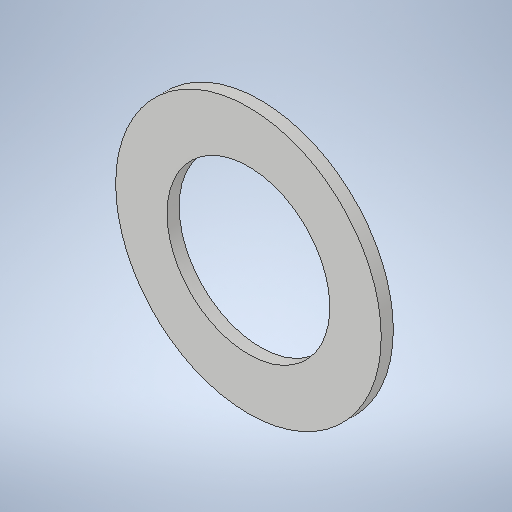
# Autodesk Inventor part: Fixierplatte_Innenring58,2mm
Saved by Autodesk Inventor 2025 (Build 290162000, 162)
## iProperties
Created: 2020-01-21
Part Number: Fixierplatte_Innenring58,2mm
Material: Generisch
Document SubType Name: Modeling
Designer: maxse
Density: 1 g/cm^3
Appearance: Vorgabe
Author: maxse
Autodesk Inventor part; units mm, degrees
(part 1 of 2)
ref_plane "YZ Plane" through (0, 0, 0) normal (1, 0, 0) x (0, 1, 0)
ref_plane "XZ Plane" through (0, 0, 0) normal (0, 1, 0) x (-1, 0, 0)
ref_plane "XY Plane" through (0, 0, 0) normal (0, 0, 1) x (1, 0, 0)
sketch "Skizze1" plane through (0, 0, 0) normal (0, 1, 0) x (-1, 0, 0)
  circle A0 centre (0, 0) radius 26.94
  circle A1 centre (0, 0) radius 43.95
  dimension "d0" = 53.88
  dimension "d1" = 87.9
  constraints: 2 centre point, 2 coincident
  measures "d0" diameter of A0
  measures "d1" diameter of A1
extrude "Extrusion1" add sketch "Skizze1" along normal blind 4
sketch "Skizze2" plane through (0, 4, 0) normal (0, 1, 0) x (1, 0, 0)
  circle A0 centre (0, 0) radius 26.94 projected
  spline S0 degree 2 poles (24.5434, -20.262) (24.7807, -19.9746) (25.3421, -19.6446) (25.6382, -19.6106) knots 0 0 0 1 2 2 2
  spline S1 degree 2 poles (25.6382, -19.6106) (25.9286, -19.5771) (26.4928, -19.7592) (26.7334, -19.9578) knots 0 0 0 1 2 2 2
  spline S2 degree 2 poles (26.7334, -19.9578) (27.0459, -20.2157) (27.2948, -20.9834) (27.1879, -21.4311) knots 0 0 0 1 2 2 2
  line L0 (27.1879, -21.4311) -> (27.2035, -21.444)
  spline S3 degree 2 poles (27.2035, -21.444) (27.6039, -21.2964) (28.2246, -21.3465) (28.5183, -21.5889) knots 0 0 0 1 2 2 2
  spline S4 degree 2 poles (28.5183, -21.5889) (28.9526, -21.9475) (28.9921, -23.0835) (28.5742, -23.5897) knots 0 0 0 1 2 2 2
  spline S5 degree 2 poles (28.5742, -23.5897) (28.1408, -24.1146) (27.0673, -24.2949) (26.6361, -23.9389) knots 0 0 0 1 2 2 2
  spline S6 degree 2 poles (26.6361, -23.9389) (26.3767, -23.7248) (26.1207, -23.0038) (26.2117, -22.6008) knots 0 0 0 1 2 2 2
  line L1 (26.2117, -22.6008) -> (26.1961, -22.5879)
  spline S7 degree 2 poles (26.1961, -22.5879) (25.7613, -22.7964) (25.025, -22.7718) (24.6688, -22.4777) knots 0 0 0 1 2 2 2
  spline S8 degree 2 poles (24.6688, -22.4777) (24.1751, -22.0702) (24.0997, -20.7995) (24.5434, -20.262) knots 0 0 0 1 2 2 2
  spline S9 degree 2 poles (25.0573, -21.9053) (25.2948, -22.1013) (25.7308, -22.146) (26.0938, -21.9991) knots 0 0 0 1 2 2 2
  spline S10 degree 2 poles (26.0938, -21.9991) (26.216, -21.9528) (26.5741, -21.7546) (26.8013, -21.6321) knots 0 0 0 1 2 2 2
  spline S11 degree 2 poles (26.8013, -21.6321) (26.8361, -21.3036) (26.6057, -20.7298) (26.3401, -20.5106) knots 0 0 0 1 2 2 2
  spline S12 degree 2 poles (26.3401, -20.5106) (25.9902, -20.2216) (25.1857, -20.2668) (24.9226, -20.5856) knots 0 0 0 1 2 2 2
  spline S13 degree 2 poles (24.9226, -20.5856) (24.6543, -20.9105) (24.7199, -21.6267) (25.0573, -21.9053) knots 0 0 0 1 2 2 2
  spline S14 degree 2 poles (27.0477, -23.4276) (27.307, -23.6417) (27.9402, -23.5812) (28.1956, -23.2718) knots 0 0 0 1 2 2 2
  spline S15 degree 2 poles (28.1956, -23.2718) (28.4277, -22.9906) (28.4151, -22.3759) (28.1495, -22.1566) knots 0 0 0 1 2 2 2
  spline S16 degree 2 poles (28.1495, -22.1566) (27.9589, -21.9993) (27.5411, -21.9644) (27.2826, -22.061) knots 0 0 0 1 2 2 2
  spline S17 degree 2 poles (27.2826, -22.061) (27.1744, -22.103) (26.7479, -22.3078) (26.5932, -22.4061) knots 0 0 0 1 2 2 2
  spline S18 degree 2 poles (26.5932, -22.4061) (26.5793, -22.7729) (26.8133, -23.2341) (27.0477, -23.4276) knots 0 0 0 1 2 2 2
  line L2 (23.8426, -27.2751) -> (22.4675, -22.7082)
  line L3 (22.4675, -22.7082) -> (22.9828, -22.2151)
  line L4 (22.9828, -22.2151) -> (24.3821, -26.9832)
  line L5 (24.3821, -26.9832) -> (26.247, -25.1988)
  line L6 (26.247, -25.1988) -> (26.6532, -25.6234)
  line L7 (26.6532, -25.6234) -> (24.3608, -27.8167)
  line L8 (24.3608, -27.8167) -> (23.8426, -27.2751)
  line L9 (19.5753, -25.2414) -> (20.2031, -24.7419)
  line L10 (20.2031, -24.7419) -> (20.7985, -25.4902)
  line L11 (20.7985, -25.4902) -> (20.1707, -25.9897)
  line L12 (20.1707, -25.9897) -> (19.5753, -25.2414)
  spline S19 degree 2 poles (17.1267, -28.864) (16.9289, -28.5626) (16.784, -27.9209) (16.8357, -27.6156) knots 0 0 0 1 2 2 2
  spline S20 degree 2 poles (16.8357, -27.6156) (16.8873, -27.3103) (17.2678, -26.7455) (17.593, -26.5321) knots 0 0 0 1 2 2 2
  spline S21 degree 2 poles (17.593, -26.5321) (17.8911, -26.3365) (18.5605, -26.0862) (18.8428, -26.0511) knots 0 0 0 1 2 2 2
  line L13 (18.8428, -26.0511) -> (19.2319, -26.6439)
  line L14 (19.2319, -26.6439) -> (19.1912, -26.6706)
  spline S22 degree 2 poles (19.1912, -26.6706) (19.0957, -26.6654) (18.7752, -26.7013) (18.594, -26.7427) knots 0 0 0 1 2 2 2
  spline S23 degree 2 poles (18.594, -26.7427) (18.3902, -26.7941) (18.0736, -26.9098) (17.9008, -27.0232) knots 0 0 0 1 2 2 2
  spline S24 degree 2 poles (17.9008, -27.0232) (17.7314, -27.1343) (17.493, -27.4653) (17.4646, -27.673) knots 0 0 0 1 2 2 2
  spline S25 degree 2 poles (17.4646, -27.673) (17.4418, -27.8672) (17.5513, -28.2703) (17.698, -28.4939) knots 0 0 0 1 2 2 2
  spline S26 degree 2 poles (17.698, -28.4939) (17.8448, -28.7175) (18.1535, -28.922) (18.3309, -28.9413) knots 0 0 0 1 2 2 2
  spline S27 degree 2 poles (18.3309, -28.9413) (18.5184, -28.9684) (18.9285, -28.8253) (19.1419, -28.6852) knots 0 0 0 1 2 2 2
  spline S28 degree 2 poles (19.1419, -28.6852) (19.3722, -28.5341) (19.7829, -28.1628) (19.9017, -28.0411) knots 0 0 0 1 2 2 2
  line L15 (19.9017, -28.0411) -> (21.3157, -30.1955)
  line L16 (21.3157, -30.1955) -> (19.0224, -31.7007)
  line L17 (19.0224, -31.7007) -> (18.7001, -31.2095)
  line L18 (18.7001, -31.2095) -> (20.4548, -30.0579)
  line L19 (20.4548, -30.0579) -> (19.7233, -28.9434)
  spline S29 degree 2 poles (19.7233, -28.9434) (19.6306, -29.0236) (19.4408, -29.1628) (19.3595, -29.2161) knots 0 0 0 1 2 2 2
  spline S30 degree 2 poles (19.3595, -29.2161) (19.0377, -29.4273) (18.525, -29.6136) (18.2195, -29.5911) knots 0 0 0 1 2 2 2
  spline S31 degree 2 poles (18.2195, -29.5911) (17.9106, -29.5709) (17.3757, -29.2434) (17.1267, -28.864) knots 0 0 0 1 2 2 2
  line L20 (11.7152, -29.7699) -> (12.6245, -31.7422)
  spline S32 degree 2 poles (12.6245, -31.7422) (12.7331, -31.9777) (12.9548, -32.3618) (13.0646, -32.4451) knots 0 0 0 1 2 2 2
  spline S33 degree 2 poles (13.0646, -32.4451) (13.1794, -32.5394) (13.4582, -32.5536) (13.6532, -32.4637) knots 0 0 0 1 2 2 2
  spline S34 degree 2 poles (13.6532, -32.4637) (13.8298, -32.3823) (14.1345, -31.9786) (14.2529, -31.6741) knots 0 0 0 1 2 2 2
  spline S35 degree 2 poles (14.2529, -31.6741) (14.2255, -31.6243) (14.1519, -31.4842) (14.1078, -31.3885) knots 0 0 0 1 2 2 2
  line L21 (14.1078, -31.3885) -> (13.073, -29.1439)
  line L22 (13.073, -29.1439) -> (13.647, -28.8793)
  line L23 (13.647, -28.8793) -> (14.5563, -30.8516)
  spline S36 degree 2 poles (14.5563, -30.8516) (14.6649, -31.0871) (14.8866, -31.4712) (14.9964, -31.5544) knots 0 0 0 1 2 2 2
  spline S37 degree 2 poles (14.9964, -31.5544) (15.1112, -31.6487) (15.39, -31.663) (15.585, -31.5731) knots 0 0 0 1 2 2 2
  spline S38 degree 2 poles (15.585, -31.5731) (15.769, -31.4882) (16.0705, -31.0681) (16.1787, -30.7996) knots 0 0 0 1 2 2 2
  line L24 (16.1787, -30.7996) -> (15.0048, -28.2533)
  line L25 (15.0048, -28.2533) -> (15.5788, -27.9887)
  line L26 (15.5788, -27.9887) -> (17.1497, -31.396)
  line L27 (17.1497, -31.396) -> (16.5757, -31.6606)
  line L28 (16.5757, -31.6606) -> (16.4027, -31.2853)
  spline S39 degree 2 poles (16.4027, -31.2853) (16.2817, -31.6133) (15.9538, -32.0634) (15.6889, -32.1855) knots 0 0 0 1 2 2 2
  spline S40 degree 2 poles (15.6889, -32.1855) (15.3872, -32.3246) (14.7926, -32.2641) (14.527, -32.0073) knots 0 0 0 1 2 2 2
  spline S41 degree 2 poles (14.527, -32.0073) (14.3997, -32.4185) (14.0441, -32.9438) (13.7571, -33.0762) knots 0 0 0 1 2 2 2
  spline S42 degree 2 poles (13.7571, -33.0762) (13.5363, -33.1779) (13.1129, -33.208) (12.9092, -33.1146) knots 0 0 0 1 2 2 2
  spline S43 degree 2 poles (12.9092, -33.1146) (12.7018, -33.0228) (12.3372, -32.6287) (12.176, -32.2792) knots 0 0 0 1 2 2 2
  line L29 (12.176, -32.2792) -> (11.1412, -30.0346)
  line L30 (11.1412, -30.0346) -> (11.7152, -29.7699)
  line L31 (6.1873, -31.3881) -> (6.7283, -33.4915)
  spline S44 degree 2 poles (6.7283, -33.4915) (6.7928, -33.7426) (6.9421, -34.1602) (7.0351, -34.2618) knots 0 0 0 1 2 2 2
  spline S45 degree 2 poles (7.0351, -34.2618) (7.1312, -34.3752) (7.4029, -34.4392) (7.6109, -34.3857) knots 0 0 0 1 2 2 2
  spline S46 degree 2 poles (7.6109, -34.3857) (7.7992, -34.3373) (8.1714, -33.9947) (8.3425, -33.7164) knots 0 0 0 1 2 2 2
  spline S47 degree 2 poles (8.3425, -33.7164) (8.3244, -33.6625) (8.2772, -33.5115) (8.251, -33.4095) knots 0 0 0 1 2 2 2
  line L32 (8.251, -33.4095) -> (7.6354, -31.0157)
  line L33 (7.6354, -31.0157) -> (8.2475, -30.8583)
  line L34 (8.2475, -30.8583) -> (8.7884, -32.9616)
  spline S48 degree 2 poles (8.7884, -32.9616) (8.853, -33.2128) (9.0023, -33.6304) (9.0953, -33.732) knots 0 0 0 1 2 2 2
  spline S49 degree 2 poles (9.0953, -33.732) (9.1914, -33.8454) (9.4631, -33.9094) (9.6711, -33.8559) knots 0 0 0 1 2 2 2
  spline S50 degree 2 poles (9.6711, -33.8559) (9.8673, -33.8054) (10.2393, -33.4462) (10.3939, -33.2014) knots 0 0 0 1 2 2 2
  line L35 (10.3939, -33.2014) -> (9.6955, -30.4859)
  line L36 (9.6955, -30.4859) -> (10.3077, -30.3285)
  line L37 (10.3077, -30.3285) -> (11.2422, -33.9622)
  line L38 (11.2422, -33.9622) -> (10.63, -34.1197)
  line L39 (10.63, -34.1197) -> (10.5271, -33.7194)
  spline S51 degree 2 poles (10.5271, -33.7194) (10.3493, -34.0203) (9.946, -34.4044) (9.6635, -34.477) knots 0 0 0 1 2 2 2
  spline S52 degree 2 poles (9.6635, -34.477) (9.3417, -34.5598) (8.7676, -34.3936) (8.5524, -34.0934) knots 0 0 0 1 2 2 2
  spline S53 degree 2 poles (8.5524, -34.0934) (8.3535, -34.475) (7.9094, -34.9281) (7.6033, -35.0068) knots 0 0 0 1 2 2 2
  spline S54 degree 2 poles (7.6033, -35.0068) (7.3678, -35.0674) (6.9459, -35.0211) (6.7623, -34.8926) knots 0 0 0 1 2 2 2
  spline S55 degree 2 poles (6.7623, -34.8926) (6.5747, -34.7651) (6.2866, -34.3121) (6.1908, -33.9393) knots 0 0 0 1 2 2 2
  line L40 (6.1908, -33.9393) -> (5.5752, -31.5455)
  line L41 (5.5752, -31.5455) -> (6.1873, -31.3881)
  spline S56 degree 2 poles (1.4176, -31.8386) (1.9313, -31.8086) (2.544, -32.3613) (2.5811, -32.9964) knots 0 0 0 1 2 2 2
  line L42 (2.5811, -32.9964) -> (2.7023, -35.0714)
  line L43 (2.7023, -35.0714) -> (3.127, -35.0466)
  line L44 (3.127, -35.0466) -> (3.1575, -35.5684)
  line L45 (3.1575, -35.5684) -> (2.7328, -35.5932)
  line L46 (2.7328, -35.5932) -> (2.7956, -36.6692)
  line L47 (2.7956, -36.6692) -> (2.1646, -36.7061)
  line L48 (2.1646, -36.7061) -> (2.1017, -35.6301)
  line L49 (2.1017, -35.6301) -> (0.9408, -35.6979)
  line L50 (0.9408, -35.6979) -> (0.9104, -35.1761)
  line L51 (0.9104, -35.1761) -> (2.0713, -35.1083)
  line L52 (2.0713, -35.1083) -> (1.9671, -33.3245)
  spline S57 degree 2 poles (1.9671, -33.3245) (1.9505, -33.0413) (1.9121, -32.731) (1.8355, -32.6016) knots 0 0 0 1 2 2 2
  spline S58 degree 2 poles (1.8355, -32.6016) (1.772, -32.4876) (1.5104, -32.3852) (1.2919, -32.3979) knots 0 0 0 1 2 2 2
  spline S59 degree 2 poles (1.2919, -32.3979) (1.1382, -32.4069) (0.8565, -32.5167) (0.7934, -32.5488) knots 0 0 0 1 2 2 2
  line L53 (0.7934, -32.5488) -> (0.757, -32.5509)
  line L54 (0.757, -32.5509) -> (0.7239, -31.9846)
  spline S60 degree 2 poles (0.7239, -31.9846) (0.8991, -31.9257) (1.2598, -31.8478) (1.4176, -31.8386) knots 0 0 0 1 2 2 2
  spline S61 degree 2 poles (-2.8919, -33.7338) (-2.8578, -32.7862) (-1.9095, -31.7865) (-1.1482, -31.8139) knots 0 0 0 1 2 2 2
  spline S62 degree 2 poles (-1.1482, -31.8139) (-0.3667, -31.8421) (0.4898, -32.9393) (0.4568, -33.8544) knots 0 0 0 1 2 2 2
  spline S63 degree 2 poles (0.4568, -33.8544) (0.423, -34.7938) (-0.5377, -35.8012) (-1.2909, -35.7741) knots 0 0 0 1 2 2 2
  spline S64 degree 2 poles (-1.2909, -35.7741) (-2.0521, -35.7467) (-2.9259, -34.6772) (-2.8919, -33.7338) knots 0 0 0 1 2 2 2
  spline S65 degree 2 poles (-2.24, -33.7573) (-2.2662, -34.4861) (-1.7613, -35.2138) (-1.2713, -35.2315) knots 0 0 0 1 2 2 2
  spline S66 degree 2 poles (-1.2713, -35.2315) (-0.7814, -35.2491) (-0.2214, -34.5598) (-0.1951, -33.8309) knots 0 0 0 1 2 2 2
  spline S67 degree 2 poles (-0.1951, -33.8309) (-0.1696, -33.1223) (-0.6778, -32.3742) (-1.1678, -32.3565) knots 0 0 0 1 2 2 2
  spline S68 degree 2 poles (-1.1678, -32.3565) (-1.6537, -32.339) (-2.214, -33.0365) (-2.24, -33.7573) knots 0 0 0 1 2 2 2
  spline S69 degree 2 poles (-8.8075, -32.3865) (-8.7288, -32.0346) (-8.3688, -31.484) (-8.1137, -31.3086) knots 0 0 0 1 2 2 2
  spline S70 degree 2 poles (-8.1137, -31.3086) (-7.8585, -31.1332) (-7.1881, -31.0134) (-6.8085, -31.0984) knots 0 0 0 1 2 2 2
  spline S71 degree 2 poles (-6.8085, -31.0984) (-6.4605, -31.1763) (-5.815, -31.4828) (-5.5933, -31.6611) knots 0 0 0 1 2 2 2
  line L55 (-5.5933, -31.6611) -> (-5.7482, -32.3531)
  line L56 (-5.7482, -32.3531) -> (-5.7957, -32.3424)
  spline S72 degree 2 poles (-5.7957, -32.3424) (-5.8584, -32.2703) (-6.1073, -32.0651) (-6.2631, -31.9638) knots 0 0 0 1 2 2 2
  spline S73 degree 2 poles (-6.2631, -31.9638) (-6.4418, -31.8532) (-6.7453, -31.7063) (-6.9469, -31.6612) knots 0 0 0 1 2 2 2
  spline S74 degree 2 poles (-6.9469, -31.6612) (-7.1446, -31.6169) (-7.5482, -31.6761) (-7.7171, -31.8002) knots 0 0 0 1 2 2 2
  spline S75 degree 2 poles (-7.7171, -31.8002) (-7.8725, -31.919) (-8.0857, -32.2782) (-8.1442, -32.5392) knots 0 0 0 1 2 2 2
  spline S76 degree 2 poles (-8.1442, -32.5392) (-8.2026, -32.8001) (-8.1346, -33.1641) (-8.0249, -33.3049) knots 0 0 0 1 2 2 2
  spline S77 degree 2 poles (-8.0249, -33.3049) (-7.914, -33.4585) (-7.5258, -33.6534) (-7.2767, -33.7091) knots 0 0 0 1 2 2 2
  spline S78 degree 2 poles (-7.2767, -33.7091) (-7.0078, -33.7693) (-6.4554, -33.8058) (-6.2854, -33.8065) knots 0 0 0 1 2 2 2
  line L57 (-6.2854, -33.8065) -> (-6.8484, -36.3212)
  line L58 (-6.8484, -36.3212) -> (-9.5252, -35.7219)
  line L59 (-9.5252, -35.7219) -> (-9.3968, -35.1486)
  line L60 (-9.3968, -35.1486) -> (-7.3487, -35.6071)
  line L61 (-7.3487, -35.6071) -> (-7.0575, -34.3063)
  spline S79 degree 2 poles (-7.0575, -34.3063) (-7.1796, -34.2955) (-7.4116, -34.2561) (-7.5065, -34.2348) knots 0 0 0 1 2 2 2
  spline S80 degree 2 poles (-7.5065, -34.2348) (-7.8821, -34.1507) (-8.3727, -33.9122) (-8.5692, -33.6772) knots 0 0 0 1 2 2 2
  spline S81 degree 2 poles (-8.5692, -33.6772) (-8.7697, -33.4413) (-8.9067, -32.8293) (-8.8075, -32.3865) knots 0 0 0 1 2 2 2
  spline S82 degree 2 poles (-11.9247, -34.4615) (-11.7527, -34.5218) (-11.3829, -34.5572) (-11.1957, -34.5499) knots 0 0 0 1 2 2 2
  spline S83 degree 2 poles (-11.1957, -34.5499) (-11.0199, -34.5386) (-10.746, -34.4801) (-10.6366, -34.4498) knots 0 0 0 1 2 2 2
  line L62 (-10.6366, -34.4498) -> (-10.5984, -34.4632)
  line L63 (-10.5984, -34.4632) -> (-10.8333, -35.1323)
  spline S84 degree 2 poles (-10.8333, -35.1323) (-11.0786, -35.1707) (-11.849, -35.1021) (-12.1663, -34.9907) knots 0 0 0 1 2 2 2
  spline S85 degree 2 poles (-12.1663, -34.9907) (-12.4875, -34.878) (-12.9197, -34.5803) (-13.0664, -34.3742) knots 0 0 0 1 2 2 2
  spline S86 degree 2 poles (-13.0664, -34.3742) (-13.2205, -34.1526) (-13.283, -33.6454) (-13.181, -33.3549) knots 0 0 0 1 2 2 2
  spline S87 degree 2 poles (-13.181, -33.3549) (-13.0441, -32.9649) (-12.3251, -32.556) (-11.9389, -32.6057) knots 0 0 0 1 2 2 2
  line L64 (-11.9389, -32.6057) -> (-11.9228, -32.5598)
  spline S88 degree 2 poles (-11.9228, -32.5598) (-12.0612, -32.4769) (-12.3531, -32.2198) (-12.4501, -32.0312) knots 0 0 0 1 2 2 2
  spline S89 degree 2 poles (-12.4501, -32.0312) (-12.5484, -31.8463) (-12.5816, -31.3537) (-12.4729, -31.0441) knots 0 0 0 1 2 2 2
  spline S90 degree 2 poles (-12.4729, -31.0441) (-12.3615, -30.7267) (-11.9544, -30.2642) (-11.6831, -30.1275) knots 0 0 0 1 2 2 2
  spline S91 degree 2 poles (-11.6831, -30.1275) (-11.4015, -29.9859) (-10.7387, -29.9694) (-10.3679, -30.0996) knots 0 0 0 1 2 2 2
  spline S92 degree 2 poles (-10.3679, -30.0996) (-10.0123, -30.2244) (-9.3769, -30.6407) (-9.1815, -30.8424) knots 0 0 0 1 2 2 2
  line L65 (-9.1815, -30.8424) -> (-9.4163, -31.5115)
  line L66 (-9.4163, -31.5115) -> (-9.4622, -31.4954)
  spline S93 degree 2 poles (-9.4622, -31.4954) (-9.61, -31.2803) (-10.1889, -30.7765) (-10.5215, -30.6598) knots 0 0 0 1 2 2 2
  spline S94 degree 2 poles (-10.5215, -30.6598) (-10.7165, -30.5913) (-11.1494, -30.5768) (-11.3291, -30.6726) knots 0 0 0 1 2 2 2
  spline S95 degree 2 poles (-11.3291, -30.6726) (-11.5049, -30.7698) (-11.7568, -31.0592) (-11.8467, -31.3154) knots 0 0 0 1 2 2 2
  spline S96 degree 2 poles (-11.8467, -31.3154) (-11.9366, -31.5715) (-11.9043, -31.9565) (-11.804, -32.099) knots 0 0 0 1 2 2 2
  spline S97 degree 2 poles (-11.804, -32.099) (-11.7038, -32.2416) (-11.3661, -32.4417) (-11.152, -32.5169) knots 0 0 0 1 2 2 2
  line L67 (-11.152, -32.5169) -> (-10.8843, -32.6108)
  line L68 (-10.8843, -32.6108) -> (-11.0682, -33.1346)
  line L69 (-11.0682, -33.1346) -> (-11.2785, -33.0608)
  spline S98 degree 2 poles (-11.2785, -33.0608) (-11.7028, -32.9118) (-12.3803, -33.1292) (-12.5159, -33.5153) knots 0 0 0 1 2 2 2
  spline S99 degree 2 poles (-12.5159, -33.5153) (-12.5789, -33.695) (-12.5312, -33.9995) (-12.4472, -34.1149) knots 0 0 0 1 2 2 2
  spline S100 degree 2 poles (-12.4472, -34.1149) (-12.3569, -34.2368) (-12.0891, -34.4037) (-11.9247, -34.4615) knots 0 0 0 1 2 2 2
  line L70 (-13.6422, -28.8827) -> (-12.9126, -29.2163)
  line L71 (-12.9126, -29.2163) -> (-13.3102, -30.086)
  line L72 (-13.3102, -30.086) -> (-14.0398, -29.7524)
  line L73 (-14.0398, -29.7524) -> (-13.6422, -28.8827)
  spline S101 degree 2 poles (-17.9809, -28.3398) (-17.8017, -28.0269) (-17.2952, -27.6072) (-16.9996, -27.515) knots 0 0 0 1 2 2 2
  spline S102 degree 2 poles (-16.9996, -27.515) (-16.704, -27.4228) (-16.0281, -27.5064) (-15.6906, -27.6997) knots 0 0 0 1 2 2 2
  spline S103 degree 2 poles (-15.6906, -27.6997) (-15.3812, -27.8769) (-14.8549, -28.3604) (-14.6958, -28.5962) knots 0 0 0 1 2 2 2
  line L74 (-14.6958, -28.5962) -> (-15.0482, -29.2115)
  line L75 (-15.0482, -29.2115) -> (-15.0904, -29.1874)
  spline S104 degree 2 poles (-15.0904, -29.1874) (-15.129, -29.0999) (-15.3062, -28.8303) (-15.4252, -28.6875) knots 0 0 0 1 2 2 2
  spline S105 degree 2 poles (-15.4252, -28.6875) (-15.5632, -28.5291) (-15.8098, -28.2991) (-15.9891, -28.1965) knots 0 0 0 1 2 2 2
  spline S106 degree 2 poles (-15.9891, -28.1965) (-16.1649, -28.0958) (-16.5679, -28.0331) (-16.766, -28.1017) knots 0 0 0 1 2 2 2
  spline S107 degree 2 poles (-16.766, -28.1017) (-16.9495, -28.1694) (-17.2593, -28.4495) (-17.3922, -28.6816) knots 0 0 0 1 2 2 2
  spline S108 degree 2 poles (-17.3922, -28.6816) (-17.5251, -28.9137) (-17.5677, -29.2815) (-17.5045, -29.4484) knots 0 0 0 1 2 2 2
  spline S109 degree 2 poles (-17.5045, -29.4484) (-17.4439, -29.6279) (-17.1306, -29.9287) (-16.9091, -30.0556) knots 0 0 0 1 2 2 2
  spline S110 degree 2 poles (-16.9091, -30.0556) (-16.67, -30.1925) (-16.153, -30.3905) (-15.9907, -30.4414) knots 0 0 0 1 2 2 2
  line L76 (-15.9907, -30.4414) -> (-17.2714, -32.6777)
  line L77 (-17.2714, -32.6777) -> (-19.6518, -31.3144)
  line L78 (-19.6518, -31.3144) -> (-19.3598, -30.8046)
  line L79 (-19.3598, -30.8046) -> (-17.5385, -31.8477)
  line L80 (-17.5385, -31.8477) -> (-16.876, -30.6909)
  spline S111 degree 2 poles (-16.876, -30.6909) (-16.9895, -30.6445) (-17.1995, -30.5383) (-17.2839, -30.49) knots 0 0 0 1 2 2 2
  spline S112 degree 2 poles (-17.2839, -30.49) (-17.6179, -30.2987) (-18.0161, -29.9259) (-18.1344, -29.6433) knots 0 0 0 1 2 2 2
  spline S113 degree 2 poles (-18.1344, -29.6433) (-18.2563, -29.3588) (-18.2064, -28.7336) (-17.9809, -28.3398) knots 0 0 0 1 2 2 2
  line L81 (-21.2389, -23.925) -> (-22.5857, -25.6287)
  spline S114 degree 2 poles (-22.5857, -25.6287) (-22.7465, -25.8322) (-22.9886, -26.2038) (-23.0131, -26.3393) knots 0 0 0 1 2 2 2
  spline S115 degree 2 poles (-23.0131, -26.3393) (-23.0452, -26.4844) (-22.9317, -26.7394) (-22.7632, -26.8726) knots 0 0 0 1 2 2 2
  spline S116 degree 2 poles (-22.7632, -26.8726) (-22.6107, -26.9932) (-22.1128, -27.0821) (-21.7877, -27.0498) knots 0 0 0 1 2 2 2
  spline S117 degree 2 poles (-21.7877, -27.0498) (-21.7557, -27.0028) (-21.664, -26.8738) (-21.5987, -26.7911) knots 0 0 0 1 2 2 2
  line L82 (-21.5987, -26.7911) -> (-20.066, -24.8521)
  line L83 (-20.066, -24.8521) -> (-19.5701, -25.2441)
  line L84 (-19.5701, -25.2441) -> (-20.9169, -26.9479)
  spline S118 degree 2 poles (-20.9169, -26.9479) (-21.0777, -27.1513) (-21.3198, -27.5229) (-21.3443, -27.6585) knots 0 0 0 1 2 2 2
  spline S119 degree 2 poles (-21.3443, -27.6585) (-21.3764, -27.8036) (-21.2629, -28.0586) (-21.0944, -28.1918) knots 0 0 0 1 2 2 2
  spline S120 degree 2 poles (-21.0944, -28.1918) (-20.9355, -28.3174) (-20.4244, -28.3961) (-20.1359, -28.371) knots 0 0 0 1 2 2 2
  line L85 (-20.1359, -28.371) -> (-18.3972, -26.1713)
  line L86 (-18.3972, -26.1713) -> (-17.9013, -26.5633)
  line L87 (-17.9013, -26.5633) -> (-20.228, -29.5067)
  line L88 (-20.228, -29.5067) -> (-20.7239, -29.1148)
  line L89 (-20.7239, -29.1148) -> (-20.4676, -28.7905)
  spline S121 degree 2 poles (-20.4676, -28.7905) (-20.8148, -28.8312) (-21.3646, -28.7426) (-21.5934, -28.5617) knots 0 0 0 1 2 2 2
  spline S122 degree 2 poles (-21.5934, -28.5617) (-21.8541, -28.3557) (-22.0693, -27.7982) (-21.9607, -27.445) knots 0 0 0 1 2 2 2
  spline S123 degree 2 poles (-21.9607, -27.445) (-22.3848, -27.5178) (-23.0143, -27.4385) (-23.2623, -27.2425) knots 0 0 0 1 2 2 2
  spline S124 degree 2 poles (-23.2623, -27.2425) (-23.453, -27.0918) (-23.6715, -26.7279) (-23.6804, -26.504) knots 0 0 0 1 2 2 2
  spline S125 degree 2 poles (-23.6804, -26.504) (-23.6925, -26.2775) (-23.5062, -25.774) (-23.2675, -25.472) knots 0 0 0 1 2 2 2
  line L90 (-23.2675, -25.472) -> (-21.7348, -23.533)
  line L91 (-21.7348, -23.533) -> (-21.2389, -23.925)
  line L92 (-25.1846, -19.7289) -> (-26.8151, -21.1636)
  spline S126 degree 2 poles (-26.8151, -21.1636) (-27.0098, -21.3349) (-27.3146, -21.657) (-27.363, -21.786) knots 0 0 0 1 2 2 2
  spline S127 degree 2 poles (-27.363, -21.786) (-27.4206, -21.923) (-27.3547, -22.1942) (-27.2128, -22.3554) knots 0 0 0 1 2 2 2
  spline S128 degree 2 poles (-27.2128, -22.3554) (-27.0843, -22.5015) (-26.6104, -22.6781) (-26.2848, -22.7047) knots 0 0 0 1 2 2 2
  spline S129 degree 2 poles (-26.2848, -22.7047) (-26.2449, -22.6642) (-26.1316, -22.5537) (-26.0525, -22.4841) knots 0 0 0 1 2 2 2
  line L93 (-26.0525, -22.4841) -> (-24.197, -20.8514)
  line L94 (-24.197, -20.8514) -> (-23.7794, -21.3259)
  line L95 (-23.7794, -21.3259) -> (-25.4099, -22.7606)
  spline S130 degree 2 poles (-25.4099, -22.7606) (-25.6046, -22.9319) (-25.9094, -23.254) (-25.9578, -23.383) knots 0 0 0 1 2 2 2
  spline S131 degree 2 poles (-25.9578, -23.383) (-26.0154, -23.52) (-25.9494, -23.7912) (-25.8076, -23.9524) knots 0 0 0 1 2 2 2
  spline S132 degree 2 poles (-25.8076, -23.9524) (-25.6737, -24.1045) (-25.185, -24.2736) (-24.8968, -24.3006) knots 0 0 0 1 2 2 2
  line L96 (-24.8968, -24.3006) -> (-22.7917, -22.4484)
  line L97 (-22.7917, -22.4484) -> (-22.3742, -22.9229)
  line L98 (-22.3742, -22.9229) -> (-25.191, -25.4015)
  line L99 (-25.191, -25.4015) -> (-25.6086, -24.9269)
  line L100 (-25.6086, -24.9269) -> (-25.2983, -24.6539)
  spline S133 degree 2 poles (-25.2983, -24.6539) (-25.6471, -24.6316) (-26.1721, -24.4459) (-26.3648, -24.2269) knots 0 0 0 1 2 2 2
  spline S134 degree 2 poles (-26.3648, -24.2269) (-26.5843, -23.9775) (-26.6961, -23.3904) (-26.5259, -23.0625) knots 0 0 0 1 2 2 2
  spline S135 degree 2 poles (-26.5259, -23.0625) (-26.9562, -23.058) (-27.5613, -22.8672) (-27.7701, -22.6299) knots 0 0 0 1 2 2 2
  spline S136 degree 2 poles (-27.7701, -22.6299) (-27.9307, -22.4474) (-28.0804, -22.0502) (-28.049, -21.8283) knots 0 0 0 1 2 2 2
  spline S137 degree 2 poles (-28.049, -21.8283) (-28.0203, -21.6033) (-27.7468, -21.1414) (-27.4578, -20.8871) knots 0 0 0 1 2 2 2
  line L101 (-27.4578, -20.8871) -> (-25.6022, -19.2544)
  line L102 (-25.6022, -19.2544) -> (-25.1846, -19.7289)
  line L103 (31.4609, 15.2601) -> (28.1091, 13.4697)
  line L104 (28.1091, 13.4697) -> (27.4336, 14.7343)
  spline S138 degree 2 poles (27.4336, 14.7343) (27.2549, 15.069) (27.1939, 15.263) knots 0 0 0 1 1 1
  spline S139 degree 2 poles (27.1939, 15.263) (27.1024, 15.5326) (27.155, 15.9876) (27.4622, 16.4144) (27.7126, 16.5481) knots 0 0 0 1 2 3 3 3
  spline S140 degree 2 poles (27.7126, 16.5481) (28.1392, 16.776) (29.0226, 16.5484) (29.4019, 15.8382) knots 0 0 0 1 2 2 2
  line L105 (29.4019, 15.8382) -> (29.8618, 14.9773)
  line L106 (29.8618, 14.9773) -> (31.2235, 15.7046)
  line L107 (31.2235, 15.7046) -> (31.4609, 15.2601)
  line L108 (29.4658, 14.7658) -> (29.0032, 15.6318)
  spline S141 degree 2 poles (29.0032, 15.6318) (28.7726, 16.0636) (28.2609, 16.2532) (27.9696, 16.0976) knots 0 0 0 1 2 2 2
  spline S142 degree 2 poles (27.9696, 16.0976) (27.7601, 15.9857) (27.5719, 15.6127) (27.6187, 15.4144) knots 0 0 0 1 2 2 2
  spline S143 degree 2 poles (27.6187, 15.4144) (27.6481, 15.2856) (27.8092, 14.9841) knots 0 0 0 1 1 1
  line L109 (27.8092, 14.9841) -> (28.2677, 14.1258)
  line L110 (28.2677, 14.1258) -> (29.4658, 14.7658)
  spline S144 degree 2 poles (28.5075, 19.6217) (28.8348, 19.5254) (29.2479, 19.2255) (29.3995, 18.9959) knots 0 0 0 1 2 2 2
  spline S145 degree 2 poles (29.3995, 18.9959) (29.65, 18.6164) (29.5483, 17.9662) (29.2606, 17.7763) knots 0 0 0 1 2 2 2
  spline S146 degree 2 poles (29.2606, 17.7763) (29.0914, 17.6646) (28.7113, 17.6358) (28.3794, 17.7706) (28.2346, 17.9006) knots 0 0 0 1 2 3 3 3
  spline S147 degree 2 poles (28.2346, 17.9006) (28.1282, 17.9935) (27.946, 18.2064) knots 0 0 0 1 1 1
  spline S148 degree 2 poles (27.946, 18.2064) (27.5792, 18.6411) (27.3551, 18.8124) knots 0 0 0 1 1 1
  spline S149 degree 2 poles (27.3551, 18.8124) (27.2737, 18.7621) (27.252, 18.7478) knots 0 0 0 1 1 1
  spline S150 degree 2 poles (27.252, 18.7478) (27.0127, 18.5898) (26.9894, 18.4148) knots 0 0 0 1 1 1
  spline S151 degree 2 poles (26.9894, 18.4148) (26.9538, 18.1796) (27.1484, 17.8847) knots 0 0 0 1 1 1
  spline S152 degree 2 poles (27.1484, 17.8847) (27.3287, 17.6115) (27.6944, 17.4781) (27.9801, 17.5764) knots 0 0 0 1 2 2 2
  line L111 (27.9801, 17.5764) -> (28.1814, 17.161)
  spline S153 degree 2 poles (28.1814, 17.161) (27.9038, 17.0506) (27.4436, 17.0905) (26.9849, 17.4332) (26.7902, 17.7281) knots 0 0 0 1 2 3 3 3
  spline S154 degree 2 poles (26.7902, 17.7281) (26.5956, 18.023) (26.4908, 18.4813) (26.5862, 18.7942) (26.7234, 18.9333) knots 0 0 0 1 2 3 3 3
  spline S155 degree 2 poles (26.7234, 18.9333) (26.8122, 19.0197) (27.0708, 19.1904) knots 0 0 0 1 1 1
  line L112 (27.0708, 19.1904) -> (27.5905, 19.5335)
  spline S156 degree 2 poles (27.5905, 19.5335) (28.132, 19.8909) (28.3861, 20.1315) (28.4712, 20.2918) knots 0 0 0 1 2 2 2
  line L113 (28.4712, 20.2918) -> (28.7392, 19.8857)
  spline S157 degree 2 poles (28.7392, 19.8857) (28.6583, 19.7455) (28.5075, 19.6217) knots 0 0 0 1 1 1
  spline S158 degree 2 poles (27.658, 19.0158) (27.8855, 18.8606) (28.2251, 18.4775) knots 0 0 0 1 1 1
  spline S159 degree 2 poles (28.2251, 18.4775) (28.4185, 18.2581) (28.6364, 18.1173) (28.875, 18.1186) (28.9765, 18.1856) knots 0 0 0 1 2 3 3 3
  spline S160 degree 2 poles (28.9765, 18.1856) (29.1312, 18.2878) (29.1843, 18.6595) (29.0343, 18.8867) knots 0 0 0 1 2 2 2
  spline S161 degree 2 poles (29.0343, 18.8867) (28.8859, 19.1115) (28.4588, 19.3327) (28.2329, 19.3016) knots 0 0 0 1 2 2 2
  spline S162 degree 2 poles (28.2329, 19.3016) (28.0585, 19.2767) (27.8023, 19.1076) knots 0 0 0 1 1 1
  line L114 (27.8023, 19.1076) -> (27.658, 19.0158)
  line L115 (28.1217, 20.7428) -> (25.9305, 19.0738)
  line L116 (25.9305, 19.0738) -> (25.676, 19.4079)
  line L117 (25.676, 19.4079) -> (26.0078, 19.6606)
  spline S163 degree 2 poles (26.0078, 19.6606) (25.6786, 19.6101) (25.3661, 19.7144) (25.2661, 19.8457) knots 0 0 0 1 2 2 2
  spline S164 degree 2 poles (25.2661, 19.8457) (25.124, 20.0323) (25.094, 20.3154) knots 0 0 0 1 1 1
  line L118 (25.094, 20.3154) -> (25.5379, 20.4496)
  spline S165 degree 2 poles (25.5379, 20.4496) (25.5608, 20.2522) (25.6644, 20.1163) knots 0 0 0 1 1 1
  spline S166 degree 2 poles (25.6644, 20.1163) (25.7574, 19.9942) (26.0505, 19.9153) (26.2111, 19.9721) knots 0 0 0 1 2 2 2
  spline S167 degree 2 poles (26.2111, 19.9721) (26.4567, 20.0608) (26.6917, 20.2398) knots 0 0 0 1 1 1
  line L119 (26.6917, 20.2398) -> (27.8391, 21.1138)
  line L120 (27.8391, 21.1138) -> (28.1217, 20.7428)
  line L121 (27.0294, 22.1421) -> (24.9105, 20.3822)
  line L122 (24.9105, 20.3822) -> (24.6125, 20.741)
  line L123 (24.6125, 20.741) -> (26.7314, 22.5008)
  line L124 (26.7314, 22.5008) -> (27.0294, 22.1421)
  line L125 (24.5183, 20.0566) -> (24.1061, 19.7142)
  line L126 (24.1061, 19.7142) -> (23.8082, 20.0729)
  line L127 (23.8082, 20.0729) -> (24.2204, 20.4153)
  line L128 (24.2204, 20.4153) -> (24.5183, 20.0566)
  line L129 (25.804, 22.3497) -> (25.4377, 22.6381)
  spline S168 degree 2 poles (25.4377, 22.6381) (25.616, 22.8548) (25.5902, 23.3169) (25.3716, 23.5526) knots 0 0 0 1 2 2 2
  spline S169 degree 2 poles (25.3716, 23.5526) (25.1529, 23.7883) (24.7469, 23.8383) (24.6174, 23.7182) knots 0 0 0 1 2 2 2
  spline S170 degree 2 poles (24.6174, 23.7182) (24.5028, 23.6118) (24.5294, 23.4468) knots 0 0 0 1 1 1
  spline S171 degree 2 poles (24.5294, 23.4468) (24.5498, 23.3354) (24.7398, 22.9901) knots 0 0 0 1 1 1
  spline S172 degree 2 poles (24.7398, 22.9901) (24.9929, 22.5257) (25.1247, 22.1067) (25.0183, 21.7275) (24.8718, 21.5915) knots 0 0 0 1 2 3 3 3
  spline S173 degree 2 poles (24.8718, 21.5915) (24.7359, 21.4655) (24.3923, 21.3759) (24.2174, 21.4111) knots 0 0 0 1 2 2 2
  spline S174 degree 2 poles (24.2174, 21.4111) (24.0831, 21.4366) (23.7463, 21.6378) (23.5986, 21.7971) knots 0 0 0 1 2 2 2
  spline S175 degree 2 poles (23.5986, 21.7971) (23.378, 22.0349) (23.1831, 22.5217) (23.2571, 22.9104) (23.4228, 23.1235) knots 0 0 0 1 2 3 3 3
  line L130 (23.4228, 23.1235) -> (23.7787, 22.8294)
  spline S176 degree 2 poles (23.7787, 22.8294) (23.6432, 22.6603) (23.672, 22.28) (23.8572, 22.0804) knots 0 0 0 1 2 2 2
  spline S177 degree 2 poles (23.8572, 22.0804) (24.0758, 21.8448) (24.4201, 21.7888) (24.5242, 21.8853) knots 0 0 0 1 2 2 2
  spline S178 degree 2 poles (24.5242, 21.8853) (24.59, 21.9464) (24.6037, 22.0381) knots 0 0 0 1 1 1
  spline S179 degree 2 poles (24.6037, 22.0381) (24.6214, 22.1297) (24.5728, 22.2545) knots 0 0 0 1 1 1
  spline S180 degree 2 poles (24.5728, 22.2545) (24.5447, 22.3232) (24.3823, 22.6387) knots 0 0 0 1 1 1
  spline S181 degree 2 poles (24.3823, 22.6387) (24.141, 23.0904) (23.9962, 23.4935) (24.0802, 23.8756) (24.2564, 24.0391) knots 0 0 0 1 2 3 3 3
  spline S182 degree 2 poles (24.2564, 24.0391) (24.4263, 24.1967) (24.913, 24.2768) (25.4292, 24.0525) (25.6499, 23.8147) knots 0 0 0 1 2 3 3 3
  spline S183 degree 2 poles (25.6499, 23.8147) (26.0143, 23.4219) (26.0714, 22.7045) (25.804, 22.3497) knots 0 0 0 1 2 2 2
  line L131 (23.353, 26.012) -> (20.9036, 23.1068)
  line L132 (20.9036, 23.1068) -> (20.5183, 23.4316)
  line L133 (20.5183, 23.4316) -> (22.6783, 25.9936)
  line L134 (22.6783, 25.9936) -> (21.2478, 27.1997)
  line L135 (21.2478, 27.1997) -> (21.5372, 27.5429)
  line L136 (21.5372, 27.5429) -> (23.353, 26.012)
  spline S184 degree 2 poles (20.4524, 26.6411) (20.0123, 26.0194) (19.4523, 25.9652) knots 0 0 0 1 1 1
  spline S185 degree 2 poles (19.4523, 25.9652) (18.9865, 25.9188) (18.5704, 26.2134) knots 0 0 0 1 1 1
  spline S186 degree 2 poles (18.5704, 26.2134) (18.1071, 26.5414) (17.9486, 27.5656) (18.3268, 28.0998) knots 0 0 0 1 2 2 2
  spline S187 degree 2 poles (18.3268, 28.0998) (18.6331, 28.5324) (19.2462, 28.8471) (19.9368, 28.7699) (20.2322, 28.5607) knots 0 0 0 1 2 3 3 3
  spline S188 degree 2 poles (20.2322, 28.5607) (20.7027, 28.2277) (20.8558, 27.2108) (20.4524, 26.6411) knots 0 0 0 1 2 2 2
  spline S189 degree 2 poles (20.0617, 26.9213) (20.3663, 27.3515) (20.295, 28.0478) (20.0113, 28.2487) knots 0 0 0 1 2 2 2
  spline S190 degree 2 poles (20.0113, 28.2487) (19.7277, 28.4495) (19.0456, 28.283) (18.7326, 27.8409) knots 0 0 0 1 2 2 2
  spline S191 degree 2 poles (18.7326, 27.8409) (18.4381, 27.4249) (18.5117, 26.7269) (18.793, 26.5277) knots 0 0 0 1 2 2 2
  spline S192 degree 2 poles (18.793, 26.5277) (19.0767, 26.3269) (19.7554, 26.4887) (20.0617, 26.9213) knots 0 0 0 1 2 2 2
  line L137 (17.1419, 30.4532) -> (16.9657, 30.1536)
  spline S193 degree 2 poles (16.9657, 30.1536) (17.3975, 30.3735) (17.8369, 30.115) knots 0 0 0 1 1 1
  spline S194 degree 2 poles (17.8369, 30.115) (18.1215, 29.9477) (18.4123, 29.3566) (18.3441, 28.6407) (18.1297, 28.2762) knots 0 0 0 1 2 3 3 3
  spline S195 degree 2 poles (18.1297, 28.2762) (17.9212, 27.9217) (17.3434, 27.482) (16.6909, 27.4524) (16.3988, 27.6242) knots 0 0 0 1 2 3 3 3
  spline S196 degree 2 poles (16.3988, 27.6242) (16.1841, 27.7504) (15.9553, 28.127) (15.9356, 28.3334) knots 0 0 0 1 2 2 2
  line L138 (15.9356, 28.3334) -> (15.2455, 27.16)
  line L139 (15.2455, 27.16) -> (14.8436, 27.3964)
  line L140 (14.8436, 27.3964) -> (16.7699, 30.6719)
  line L141 (16.7699, 30.6719) -> (17.1419, 30.4532)
  spline S197 degree 2 poles (17.7153, 28.5199) (17.984, 28.9768) (17.8652, 29.6548) (17.6031, 29.809) knots 0 0 0 1 2 2 2
  spline S198 degree 2 poles (17.6031, 29.809) (17.341, 29.9632) (16.7175, 29.7485) (16.4576, 29.3066) knots 0 0 0 1 2 2 2
  spline S199 degree 2 poles (16.4576, 29.3066) (16.1713, 28.8198) (16.2771, 28.1427) (16.5517, 27.9812) knots 0 0 0 1 2 2 2
  spline S200 degree 2 poles (16.5517, 27.9812) (16.8213, 27.8226) (17.4392, 28.0506) (17.7153, 28.5199) knots 0 0 0 1 2 2 2
  line L142 (16.1228, 31.0024) -> (14.8898, 28.5394)
  line L143 (14.8898, 28.5394) -> (14.5142, 28.7274)
  line L144 (14.5142, 28.7274) -> (14.7009, 29.1003)
  spline S201 degree 2 poles (14.7009, 29.1003) (14.4275, 28.9101) (14.1011, 28.8662) (13.9535, 28.9401) knots 0 0 0 1 2 2 2
  spline S202 degree 2 poles (13.9535, 28.9401) (13.7437, 29.0451) (13.5923, 29.2861) knots 0 0 0 1 1 1
  line L145 (13.5923, 29.2861) -> (13.9318, 29.602)
  spline S203 degree 2 poles (13.9318, 29.602) (14.0392, 29.4348) (14.192, 29.3584) knots 0 0 0 1 1 1
  spline S204 degree 2 poles (14.192, 29.3584) (14.3293, 29.2896) (14.6272, 29.3478) (14.7464, 29.4695) knots 0 0 0 1 2 2 2
  spline S205 degree 2 poles (14.7464, 29.4695) (14.9279, 29.6572) (15.0601, 29.9214) knots 0 0 0 1 1 1
  line L146 (15.0601, 29.9214) -> (15.7058, 31.2112)
  line L147 (15.7058, 31.2112) -> (16.1228, 31.0024)
  spline S206 degree 2 poles (14.164, 30.4537) (13.8698, 29.7512) (13.335, 29.5764) knots 0 0 0 1 1 1
  spline S207 degree 2 poles (13.335, 29.5764) (12.8904, 29.4297) (12.4202, 29.6266) knots 0 0 0 1 1 1
  spline S208 degree 2 poles (12.4202, 29.6266) (11.8966, 29.846) (11.519, 30.8111) (11.7719, 31.4149) knots 0 0 0 1 2 2 2
  spline S209 degree 2 poles (11.7719, 31.4149) (11.9767, 31.9038) (12.5066, 32.3444) (13.1974, 32.4193) (13.5314, 32.2794) knots 0 0 0 1 2 3 3 3
  spline S210 degree 2 poles (13.5314, 32.2794) (14.063, 32.0567) (14.4337, 31.0976) (14.164, 30.4537) knots 0 0 0 1 2 2 2
  spline S211 degree 2 poles (13.7217, 30.6422) (13.9254, 31.1284) (13.7042, 31.7925) (13.3837, 31.9268) knots 0 0 0 1 2 2 2
  spline S212 degree 2 poles (13.3837, 31.9268) (13.0631, 32.061) (12.4336, 31.7501) (12.2243, 31.2505) knots 0 0 0 1 2 2 2
  spline S213 degree 2 poles (12.2243, 31.2505) (12.0274, 30.7803) (12.2512, 30.1151) (12.5691, 29.9819) knots 0 0 0 1 2 2 2
  spline S214 degree 2 poles (12.5691, 29.9819) (12.8896, 29.8477) (13.5169, 30.1533) (13.7217, 30.6422) knots 0 0 0 1 2 2 2
  line L148 (11.8039, 32.905) -> (10.9578, 30.2837)
  line L149 (10.9578, 30.2837) -> (10.5581, 30.4127)
  line L150 (10.5581, 30.4127) -> (10.6782, 30.7848)
  spline S215 degree 2 poles (10.6782, 30.7848) (10.25, 30.4483) (9.707, 30.6236) knots 0 0 0 1 1 1
  spline S216 degree 2 poles (9.707, 30.6236) (9.47, 30.7001) (9.1282, 30.9991) (9.0188, 31.3388) (9.0416, 31.5414) knots 0 0 0 1 2 3 3 3
  spline S217 degree 2 poles (9.0416, 31.5414) (9.0568, 31.6735) (9.1564, 31.9822) knots 0 0 0 1 1 1
  line L151 (9.1564, 31.9822) -> (9.676, 33.5918)
  line L152 (9.676, 33.5918) -> (10.1198, 33.4486)
  line L153 (10.1198, 33.4486) -> (9.6055, 31.8555)
  spline S218 degree 2 poles (9.6055, 31.8555) (9.5183, 31.5853) (9.5359, 31.2814) (9.7461, 31.037) (9.9253, 30.9792) knots 0 0 0 1 2 3 3 3
  spline S219 degree 2 poles (9.9253, 30.9792) (10.2092, 30.8875) (10.7364, 31.1161) (10.8984, 31.6177) knots 0 0 0 1 2 2 2
  line L154 (10.8984, 31.6177) -> (11.3601, 33.0482)
  line L155 (11.3601, 33.0482) -> (11.8039, 32.905)
  line L156 (4.3908, 30.8446) -> (3.8944, 30.9314)
  line L157 (3.8944, 30.9314) -> (4.2723, 33.094)
  spline S220 degree 2 poles (4.2723, 33.094) (4.3711, 33.6589) (4.7407, 34.2765) (5.4811, 34.5763) (6.0232, 34.4816) knots 0 0 0 1 2 3 3 3
  spline S221 degree 2 poles (6.0232, 34.4816) (6.5482, 34.3899) (7.1553, 33.9103) (7.3205, 33.1729) (7.2167, 32.5794) knots 0 0 0 1 2 3 3 3
  line L158 (7.2167, 32.5794) -> (6.8388, 30.4168)
  line L159 (6.8388, 30.4168) -> (6.3424, 30.5036)
  line L160 (6.3424, 30.5036) -> (6.7198, 32.6634)
  spline S222 degree 2 poles (6.7198, 32.6634) (6.8046, 33.1484) (6.7056, 33.642) (6.3072, 33.9704) (5.9877, 34.0262) knots 0 0 0 1 2 3 3 3
  spline S223 degree 2 poles (5.9877, 34.0262) (5.4428, 34.1214) (4.8909, 33.7063) (4.7683, 33.0044) knots 0 0 0 1 2 2 2
  line L161 (4.7683, 33.0044) -> (4.3908, 30.8446)
  line L162 (3.7743, 34.7538) -> (3.5653, 32.0073)
  line L163 (3.5653, 32.0073) -> (3.1465, 32.0392)
  line L164 (3.1465, 32.0392) -> (3.1762, 32.429)
  spline S224 degree 2 poles (3.1762, 32.429) (2.8386, 32.0016) (2.2697, 32.0449) knots 0 0 0 1 1 1
  spline S225 degree 2 poles (2.2697, 32.0449) (2.0213, 32.0638) (1.6191, 32.2745) (1.4332, 32.5792) (1.4079, 32.7815) knots 0 0 0 1 2 3 3 3
  spline S226 degree 2 poles (1.4079, 32.7815) (1.3918, 32.9135) (1.4164, 33.2369) knots 0 0 0 1 1 1
  line L165 (1.4164, 33.2369) -> (1.5448, 34.9235)
  line L166 (1.5448, 34.9235) -> (2.0098, 34.8881)
  line L167 (2.0098, 34.8881) -> (1.8827, 33.2188)
  spline S227 degree 2 poles (1.8827, 33.2188) (1.8612, 32.9358) (1.9494, 32.6444) (2.211, 32.4561) (2.3987, 32.4418) knots 0 0 0 1 2 3 3 3
  spline S228 degree 2 poles (2.3987, 32.4418) (2.6961, 32.4191) (3.1553, 32.7647) (3.1953, 33.2903) knots 0 0 0 1 2 2 2
  line L168 (3.1953, 33.2903) -> (3.3094, 34.7892)
  line L169 (3.3094, 34.7892) -> (3.7743, 34.7538)
  line L170 (0.8268, 34.931) -> (0.7802, 32.177)
  line L171 (0.7802, 32.177) -> (0.3139, 32.1849)
  line L172 (0.3139, 32.1849) -> (0.3605, 34.9389)
  line L173 (0.3605, 34.9389) -> (0.8268, 34.931)
  line L174 (0.7716, 31.6673) -> (0.7625, 31.1316)
  line L175 (0.7625, 31.1316) -> (0.2963, 31.1394)
  line L176 (0.2963, 31.1394) -> (0.3053, 31.6752)
  line L177 (0.3053, 31.6752) -> (0.7716, 31.6673)
  line L178 (-1.1071, 34.9231) -> (0.0393, 32.2103)
  line L179 (0.0393, 32.2103) -> (-0.4527, 32.1916)
  line L180 (-0.4527, 32.1916) -> (-1.1057, 33.8189)
  spline S229 degree 2 poles (-1.1057, 33.8189) (-1.2114, 34.0815) (-1.3033, 34.365) knots 0 0 0 1 1 1
  spline S230 degree 2 poles (-1.3033, 34.365) (-1.3558, 34.1456) (-1.4542, 33.8346) knots 0 0 0 1 1 1
  line L181 (-1.4542, 33.8346) -> (-2.0011, 32.1328)
  line L182 (-2.0011, 32.1328) -> (-2.4816, 32.1146)
  line L183 (-2.4816, 32.1146) -> (-1.5441, 34.9065)
  line L184 (-1.5441, 34.9065) -> (-1.1071, 34.9231)
  line L185 (-4.7658, 33.7242) -> (-5.2533, 33.7276)
  spline S231 degree 2 poles (-5.2533, 33.7276) (-5.1881, 34.1611) (-4.6304, 34.6969) (-4.1558, 34.7532) knots 0 0 0 1 2 2 2
  spline S232 degree 2 poles (-4.1558, 34.7532) (-3.5547, 34.8246) (-2.7652, 34.1687) (-2.6863, 33.5043) knots 0 0 0 1 2 2 2
  spline S233 degree 2 poles (-2.6863, 33.5043) (-2.6044, 32.8141) (-3.2243, 31.9675) (-3.7909, 31.9003) knots 0 0 0 1 2 2 2
  spline S234 degree 2 poles (-3.7909, 31.9003) (-4.3374, 31.8354) (-5.1222, 32.5006) (-5.2024, 33.1765) knots 0 0 0 1 2 2 2
  spline S235 degree 2 poles (-5.2024, 33.1765) (-5.2072, 33.2168) (-5.2142, 33.3005) knots 0 0 0 1 1 1
  line L186 (-5.2142, 33.3005) -> (-3.175, 33.5426)
  spline S236 degree 2 poles (-3.175, 33.5426) (-3.2545, 33.9911) (-3.7685, 34.4142) (-4.1108, 34.3736) knots 0 0 0 1 2 2 2
  spline S237 degree 2 poles (-4.1108, 34.3736) (-4.3668, 34.3432) (-4.6942, 34.0302) (-4.7658, 33.7242) knots 0 0 0 1 2 2 2
  line L187 (-3.1559, 33.1598) -> (-4.6831, 32.9786)
  spline S238 degree 2 poles (-4.6831, 32.9786) (-4.6105, 32.6372) (-4.4459, 32.4788) knots 0 0 0 1 1 1
  spline S239 degree 2 poles (-4.4459, 32.4788) (-4.1927, 32.2376) (-3.8389, 32.2796) knots 0 0 0 1 1 1
  spline S240 degree 2 poles (-3.8389, 32.2796) (-3.5196, 32.3175) (-3.1362, 32.7976) (-3.1559, 33.1598) knots 0 0 0 1 2 2 2
  line L188 (-5.9194, 34.4391) -> (-5.411, 31.732)
  line L189 (-5.411, 31.732) -> (-5.8238, 31.6545)
  line L190 (-5.8238, 31.6545) -> (-5.9008, 32.0644)
  spline S241 degree 2 poles (-5.9008, 32.0644) (-6.0033, 31.7475) (-6.2367, 31.5151) (-6.399, 31.4846) knots 0 0 0 1 2 2 2
  spline S242 degree 2 poles (-6.399, 31.4846) (-6.6295, 31.4413) (-6.8959, 31.5416) knots 0 0 0 1 1 1
  line L191 (-6.8959, 31.5416) -> (-6.8167, 31.9985)
  spline S243 degree 2 poles (-6.8167, 31.9985) (-6.63, 31.9304) (-6.4621, 31.962) knots 0 0 0 1 1 1
  spline S244 degree 2 poles (-6.4621, 31.962) (-6.3112, 31.9903) (-6.1092, 32.2169) (-6.0879, 32.3859) knots 0 0 0 1 2 2 2
  spline S245 degree 2 poles (-6.0879, 32.3859) (-6.057, 32.6451) (-6.1115, 32.9355) knots 0 0 0 1 1 1
  line L192 (-6.1115, 32.9355) -> (-6.3777, 34.3531)
  line L193 (-6.3777, 34.3531) -> (-5.9194, 34.4391)
  line L194 (-7.2746, 33.3532) -> (-7.7031, 33.1696)
  spline S246 degree 2 poles (-7.7031, 33.1696) (-7.8081, 33.4298) (-8.2261, 33.6284) (-8.5377, 33.5492) knots 0 0 0 1 2 2 2
  spline S247 degree 2 poles (-8.5377, 33.5492) (-8.8493, 33.47) (-9.0875, 33.1375) (-9.044, 32.9663) knots 0 0 0 1 2 2 2
  spline S248 degree 2 poles (-9.044, 32.9663) (-9.0055, 32.8147) (-8.8479, 32.7591) knots 0 0 0 1 1 1
  spline S249 degree 2 poles (-8.8479, 32.7591) (-8.7403, 32.7237) (-8.3462, 32.7252) knots 0 0 0 1 1 1
  spline S250 degree 2 poles (-8.3462, 32.7252) (-7.8173, 32.7252) (-7.3863, 32.6405) (-7.1042, 32.3655) (-7.055, 32.1718) knots 0 0 0 1 2 3 3 3
  spline S251 degree 2 poles (-7.055, 32.1718) (-7.0093, 31.9922) (-7.0951, 31.6476) (-7.2098, 31.5109) knots 0 0 0 1 2 2 2
  spline S252 degree 2 poles (-7.2098, 31.5109) (-7.2965, 31.4052) (-7.6343, 31.2058) (-7.8448, 31.1523) knots 0 0 0 1 2 2 2
  spline S253 degree 2 poles (-7.8448, 31.1523) (-8.1592, 31.0724) (-8.68, 31.1342) (-8.9858, 31.3852) (-9.0936, 31.6328) knots 0 0 0 1 2 3 3 3
  line L195 (-9.0936, 31.6328) -> (-8.665, 31.8045)
  spline S254 degree 2 poles (-8.665, 31.8045) (-8.5814, 31.6046) (-8.2337, 31.4479) (-7.9699, 31.515) knots 0 0 0 1 2 2 2
  spline S255 degree 2 poles (-7.9699, 31.515) (-7.6583, 31.5942) (-7.4444, 31.8697) (-7.4794, 32.0072) knots 0 0 0 1 2 2 2
  spline S256 degree 2 poles (-7.4794, 32.0072) (-7.5015, 32.0942) (-7.5755, 32.1501) knots 0 0 0 1 1 1
  spline S257 degree 2 poles (-7.5755, 32.1501) (-7.6473, 32.2096) (-7.7802, 32.2266) knots 0 0 0 1 1 1
  spline S258 degree 2 poles (-7.7802, 32.2266) (-7.854, 32.2347) (-8.2088, 32.2432) knots 0 0 0 1 1 1
  spline S259 degree 2 poles (-8.2088, 32.2432) (-8.7209, 32.2475) (-9.144, 32.3133) (-9.4394, 32.5699) (-9.4986, 32.8029) knots 0 0 0 1 2 3 3 3
  spline S260 degree 2 poles (-9.4986, 32.8029) (-9.5557, 33.0275) (-9.3931, 33.4932) (-8.9491, 33.8391) (-8.6347, 33.919) knots 0 0 0 1 2 3 3 3
  spline S261 degree 2 poles (-8.6347, 33.919) (-8.1154, 34.051) (-7.4581, 33.7578) (-7.2746, 33.3532) knots 0 0 0 1 2 2 2
  line L196 (-10.2256, 33.411) -> (-9.4017, 30.7827)
  line L197 (-9.4017, 30.7827) -> (-9.8467, 30.6432)
  line L198 (-9.8467, 30.6432) -> (-10.6705, 33.2716)
  line L199 (-10.6705, 33.2716) -> (-10.2256, 33.411)
  line L200 (-9.2492, 30.2963) -> (-9.089, 29.785)
  line L201 (-9.089, 29.785) -> (-9.5339, 29.6455)
  line L202 (-9.5339, 29.6455) -> (-9.6942, 30.1568)
  line L203 (-9.6942, 30.1568) -> (-9.2492, 30.2963)
  line L204 (-12.1624, 32.3157) -> (-12.364, 32.6836)
  spline S262 degree 2 poles (-12.364, 32.6836) (-12.192, 32.7878) (-12.0446, 32.8402) knots 0 0 0 1 1 1
  spline S263 degree 2 poles (-12.0446, 32.8402) (-11.8072, 32.9247) (-11.4882, 32.866) (-11.2944, 32.6583) (-11.1536, 32.2626) knots 0 0 0 1 2 3 3 3
  line L205 (-11.1536, 32.2626) -> (-10.6218, 30.7672)
  line L206 (-10.6218, 30.7672) -> (-10.297, 30.8826)
  line L207 (-10.297, 30.8826) -> (-10.1757, 30.5415)
  line L208 (-10.1757, 30.5415) -> (-10.5004, 30.426)
  line L209 (-10.5004, 30.426) -> (-10.2723, 29.7848)
  line L210 (-10.2723, 29.7848) -> (-10.6176, 29.3638)
  line L211 (-10.6176, 29.3638) -> (-10.9398, 30.2698)
  line L212 (-10.9398, 30.2698) -> (-11.3791, 30.1135)
  line L213 (-11.3791, 30.1135) -> (-11.5005, 30.4546)
  line L214 (-11.5005, 30.4546) -> (-11.0611, 30.6109)
  line L215 (-11.0611, 30.6109) -> (-11.6017, 32.1309)
  spline S264 degree 2 poles (-11.6017, 32.1309) (-11.6687, 32.3192) (-11.7539, 32.4118) (-11.8799, 32.4377) (-11.9782, 32.4028) knots 0 0 0 1 2 3 3 3
  spline S265 degree 2 poles (-11.9782, 32.4028) (-12.0491, 32.3775) (-12.1624, 32.3157) knots 0 0 0 1 1 1
  spline S266 degree 2 poles (-14.2504, 31.5375) (-14.0976, 31.8425) (-13.7291, 32.1959) (-13.4762, 32.3043) knots 0 0 0 1 2 2 2
  spline S267 degree 2 poles (-13.4762, 32.3043) (-13.0583, 32.4835) (-12.4365, 32.2679) (-12.3007, 31.9511) knots 0 0 0 1 2 2 2
  spline S268 degree 2 poles (-12.3007, 31.9511) (-12.2208, 31.7648) (-12.2599, 31.3856) (-12.4515, 31.0829) (-12.6052, 30.9634) knots 0 0 0 1 2 3 3 3
  spline S269 degree 2 poles (-12.6052, 30.9634) (-12.7154, 30.8752) (-12.9573, 30.7337) knots 0 0 0 1 1 1
  spline S270 degree 2 poles (-12.9573, 30.7337) (-13.4501, 30.4499) (-13.6585, 30.2597) knots 0 0 0 1 1 1
  spline S271 degree 2 poles (-13.6585, 30.2597) (-13.6235, 30.1707) (-13.6132, 30.1468) knots 0 0 0 1 1 1
  spline S272 degree 2 poles (-13.6132, 30.1468) (-13.5003, 29.8832) (-13.3322, 29.8293) knots 0 0 0 1 1 1
  spline S273 degree 2 poles (-13.3322, 29.8293) (-13.107, 29.7525) (-12.7822, 29.8917) knots 0 0 0 1 1 1
  spline S274 degree 2 poles (-12.7822, 29.8917) (-12.4814, 30.0207) (-12.2852, 30.3569) (-12.3313, 30.6554) knots 0 0 0 1 2 2 2
  line L216 (-12.3313, 30.6554) -> (-11.8867, 30.7798)
  spline S275 degree 2 poles (-11.8867, 30.7798) (-11.8274, 30.487) (-11.9482, 30.0413) (-12.3669, 29.6506) (-12.6917, 29.5114) knots 0 0 0 1 2 3 3 3
  spline S276 degree 2 poles (-12.6917, 29.5114) (-13.0164, 29.3722) (-13.4861, 29.3504) (-13.7771, 29.4998) (-13.8897, 29.6596) knots 0 0 0 1 2 3 3 3
  spline S277 degree 2 poles (-13.8897, 29.6596) (-13.9589, 29.7622) (-14.081, 30.0471) knots 0 0 0 1 1 1
  line L217 (-14.081, 30.0471) -> (-14.3264, 30.6194)
  spline S278 degree 2 poles (-14.3264, 30.6194) (-14.582, 31.2157) (-14.7737, 31.5085) (-14.9164, 31.6207) knots 0 0 0 1 2 2 2
  line L218 (-14.9164, 31.6207) -> (-14.4692, 31.8124)
  spline S279 degree 2 poles (-14.4692, 31.8124) (-14.3455, 31.7078) (-14.2504, 31.5375) knots 0 0 0 1 1 1
  spline S280 degree 2 poles (-13.805, 30.594) (-13.6118, 30.7903) (-13.1745, 31.0565) knots 0 0 0 1 1 1
  spline S281 degree 2 poles (-13.1745, 31.0565) (-12.9243, 31.2079) (-12.7471, 31.3973) (-12.706, 31.6324) (-12.754, 31.7442) knots 0 0 0 1 2 3 3 3
  spline S282 degree 2 poles (-12.754, 31.7442) (-12.827, 31.9145) (-13.1834, 32.0328) (-13.4336, 31.9255) knots 0 0 0 1 2 2 2
  spline S283 degree 2 poles (-13.4336, 31.9255) (-13.6812, 31.8194) (-13.9747, 31.4383) (-13.9842, 31.2104) knots 0 0 0 1 2 2 2
  spline S284 degree 2 poles (-13.9842, 31.2104) (-13.9906, 31.0344) (-13.8697, 30.7522) knots 0 0 0 1 1 1
  line L219 (-13.8697, 30.7522) -> (-13.805, 30.594)
  line L220 (-11.9261, 29.5339) -> (-11.7173, 29.0468)
  line L221 (-11.7173, 29.0468) -> (-12.1645, 28.8551)
  line L222 (-12.1645, 28.8551) -> (-12.3733, 29.3422)
  line L223 (-12.3733, 29.3422) -> (-11.9261, 29.5339)
  line L224 (-12.8152, 29.1528) -> (-12.6064, 28.6656)
  line L225 (-12.6064, 28.6656) -> (-13.0536, 28.4739)
  line L226 (-13.0536, 28.4739) -> (-13.2624, 28.961)
  line L227 (-13.2624, 28.961) -> (-12.8152, 29.1528)
  line L228 (-16.1455, 30.5213) -> (-16.3919, 30.8608)
  spline S285 degree 2 poles (-16.3919, 30.8608) (-16.2345, 30.9859) (-16.0949, 31.0565) knots 0 0 0 1 1 1
  spline S286 degree 2 poles (-16.0949, 31.0565) (-15.8701, 31.1703) (-15.5461, 31.1524) (-15.3277, 30.9707) (-15.1381, 30.596) knots 0 0 0 1 2 3 3 3
  line L229 (-15.1381, 30.596) -> (-14.4217, 29.1797)
  line L230 (-14.4217, 29.1797) -> (-14.1141, 29.3353)
  line L231 (-14.1141, 29.3353) -> (-13.9507, 29.0122)
  line L232 (-13.9507, 29.0122) -> (-14.2582, 28.8566)
  line L233 (-14.2582, 28.8566) -> (-13.951, 28.2493)
  line L234 (-13.951, 28.2493) -> (-14.2403, 27.7881)
  line L235 (-14.2403, 27.7881) -> (-14.6743, 28.6461)
  line L236 (-14.6743, 28.6461) -> (-15.0905, 28.4357)
  line L237 (-15.0905, 28.4357) -> (-15.2539, 28.7587)
  line L238 (-15.2539, 28.7587) -> (-14.8378, 28.9692)
  line L239 (-14.8378, 28.9692) -> (-15.566, 30.4088)
  spline S287 degree 2 poles (-15.566, 30.4088) (-15.6562, 30.5871) (-15.7524, 30.6682) (-15.8807, 30.678) (-15.9737, 30.6309) knots 0 0 0 1 2 3 3 3
  spline S288 degree 2 poles (-15.9737, 30.6309) (-16.0409, 30.5969) (-16.1455, 30.5213) knots 0 0 0 1 1 1
  line L240 (-17.2607, 29.0053) -> (-17.6351, 28.7102)